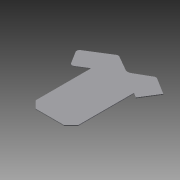
# Autodesk Inventor part: Boilermake_PCBMechanicalOverlay
Saved by Autodesk Inventor 2014 (Build 180170000, 170)
## iProperties
Created: 2014-09-13
Part Number: Boilermake_PCBMechanicalOverlay
Material: Generic
Document SubType Name: Modeling
Designer: Leeroy
Density: 1 g/cm^3
Appearance: Default
Author: Leeroy
Autodesk Inventor part; units mm, degrees
ref_plane "YZ Plane" through (0, 0, 0) normal (1, 0, 0) x (0, 1, 0)
ref_plane "XZ Plane" through (0, 0, 0) normal (0, 1, 0) x (-1, 0, 0)
ref_plane "XY Plane" through (0, 0, 0) normal (0, 0, 1) x (1, 0, 0)
sketch "Sketch1" plane through (0, 0, 0) normal (0, 0, 1) x (1, 0, 0)
  line L0 (19.7536, 18.501) -> (19.7536, -51.499)
  line L1 (-40.2464, -51.499) -> (-40.2464, 18.501)
  line L2 (-40.2464, -51.499) -> (-30.2464, -61.499)
  line L3 (-30.2464, -61.499) -> (9.7536, -61.499)
  line L4 (9.7536, -61.499) -> (19.7536, -51.499)
  line L5 (5.9033, -42.3953) -> (-35.9604, 24.6005)
  line L6 (-41.4722, 25.873) -> (-55.041, 17.3943)
  line L7 (-60.5529, 18.6668) -> (-71.151, 35.6275)
  line L8 (8.6592, -43.0315) -> (13.7475, -39.852)
  line L9 (14.3837, -37.0961) -> (-27.4799, 29.8997)
  line L10 (-26.2074, 35.4116) -> (-14.9119, 42.4698)
  line L11 (-15.0424, 49.3323) -> (-34.727, 60.6155)
  line L12 (-38.8359, 60.5374) -> (-69.8786, 41.1398)
  arc A0 (-34.727, 60.6155) -> (-38.8359, 60.5374) centre (-36.7162, 57.1452) ccw
  arc A1 (-14.9119, 42.4698) -> (-15.0424, 49.3323) centre (-17.0316, 45.8619) ccw
  arc A2 (-35.9604, 24.6005) -> (-41.4722, 25.873) centre (-39.3526, 22.4808) ccw
  arc A3 (-26.2074, 35.4116) -> (-27.4799, 29.8997) centre (-24.0877, 32.0194) ccw
  arc A4 (5.9033, -42.3953) -> (8.6592, -43.0315) centre (7.5994, -41.3354) ccw
  arc A5 (13.7475, -39.852) -> (14.3837, -37.0961) centre (12.6876, -38.1559) ccw
  line L13 (-26.3961, -42.3953) -> (15.4675, 24.6005)
  line L14 (20.9794, 25.873) -> (34.5482, 17.3943)
  line L15 (40.3411, 19.095) -> (50.6682, 35.6217)
  line L16 (-29.152, -43.0315) -> (-34.2403, -39.852)
  line L17 (-34.8766, -37.0961) -> (6.9871, 29.8997)
  line L18 (5.7136, 35.4098) -> (-5.5789, 42.4725)
  line L19 (-5.4504, 49.3323) -> (14.2435, 60.6103)
  line L20 (18.3431, 60.5374) -> (49.3859, 41.1397)
  arc A6 (18.3431, 60.5374) -> (14.2435, 60.6103) centre (16.2322, 57.1397) ccw
  arc A7 (-5.4504, 49.3323) -> (-5.5789, 42.4725) centre (-3.4579, 45.8638) ccw
  arc A8 (20.9794, 25.873) -> (15.4675, 24.6005) centre (18.8597, 22.4808) ccw
  arc A9 (6.9871, 29.8997) -> (5.7136, 35.4098) centre (3.5938, 32.0177) ccw
  arc A10 (-29.152, -43.0315) -> (-26.3961, -42.3953) centre (-28.0922, -41.3354) ccw
  arc A11 (-34.8766, -37.0961) -> (-34.2403, -39.852) centre (-33.1805, -38.1559) ccw
  arc A12 (-15.0424, 49.3323) -> (-5.4504, 49.3323) centre (-10.2464, 55.8144) ccw
  circle A13 centre (-10.2464, -7.115) radius 26
  circle A14 centre (-10.2464, -7.115) radius 20
  line L21 (-40.2464, 18.501) -> (-40.2464, 26.3797)
  line L22 (19.7536, 18.501) -> (19.7536, 26.3797)
  line L23 (-60.5529, 18.6668) -> (-60.5529, 18.6668)
  line L24 (-55.041, 17.3943) -> (-55.041, 17.3943)
  line L25 (-69.8786, 41.1398) -> (-69.8787, 41.1397)
  line L26 (-71.1513, 35.6278) -> (-71.151, 35.6275)
  arc A15 (-69.8787, 41.1397) -> (-71.1513, 35.6278) centre (-67.7591, 37.7475) ccw
  arc A16 (-60.5529, 18.6668) -> (-55.041, 17.3943) centre (-57.1607, 20.7865) ccw
  line L27 (49.3957, 41.1336) -> (49.3859, 41.1397)
  line L28 (50.6682, 35.6217) -> (50.6682, 35.6217)
  line L29 (34.5482, 17.3943) -> (34.5579, 17.3883)
  line L30 (40.3411, 19.095) -> (40.0698, 18.6608)
  arc A17 (34.5579, 17.3883) -> (40.0698, 18.6608) centre (36.6776, 20.7804) ccw
  arc A18 (50.6682, 35.6217) -> (49.3957, 41.1336) centre (47.276, 37.7414) ccw
  point P0 (0, 0)
  point P1 (-9.2464, 46.01)
  point P2 (-36.8049, 61.8065)
  point P3 (-20.4928, 0)
  point P4 (-11.243, 46.015)
  point P5 (16.3218, 61.8004)
  dimension "d0" = 70
  dimension "d1" = 135
  dimension "d2" = 135
  dimension "d3" = 10
  dimension "d4" = 10
  dimension "d5" = 40
  dimension "d6" = 10
  dimension "d7" = 85
  dimension "d8" = 24
  dimension "d9" = 24
  dimension "d10" = 28
  dimension "d11" = 43
  dimension "d13" = 2
  dimension "d14" = 31
  dimension "d15" = 32
  dimension "d19" = 70
  dimension "d21" = 52
  dimension "d22" = 40
  dimension "d43" = 8.0635
  dimension "d66" = 54.384
  dimension "d74" = 4
  dimension "d75" = 4
  dimension "d77" = 43
  dimension "d78" = 85
  dimension "d79" = 4
  constraints: 62 end point, 37 point on circle, 20 tangent, 19 centre point, 11 perpendicular, 9 point on line, 6 equal radius, 6 parallel, 3 collinear, 1 coincident, 1 vertical
  measures "d0" distance of L1.start L1.end
  measures "d1" angle of L1 L2
  measures "d2" angle of L4 L0
  measures "d3" horizontal distance of L1.start L2.end
  measures "d4" horizontal distance of L3.end L0.end
  measures "d5" distance of L2.end L3.end
  measures "d6" distance between parallel lines of L9 L5
  measures "d7" distance between parallel lines of L8 L6
  measures "d8" distance between parallel lines of L5 L7
  measures "d9" distance from line of point (-9.246, 46.01) L9
  measures "d10" distance between parallel lines of L12 L6
  measures "d11" distance from line of point (-36.805, 61.807) L7
  measures "d13" radius of A4
  measures "d14" distance from line of L1 point (-9.246, 46.01)
  measures "d15" angle of L1 L5
  measures "d19" distance of L0.start L0.end
  measures "d21" diameter of A13
  measures "d22" diameter of A14
  measures "d43" radius of A12
  measures "d66" distance from line of A13.centre L3
  measures "d74" radius of A3
  measures "d75" radius of A15
  measures "d77" distance from line of point (16.322, 61.8) L15
  measures "d78" distance between parallel lines of L16 L14
  measures "d79" radius of A17
extrude "Extrusion2" add sketch "Sketch1" along normal blind 1
sketch "Sketch11" plane through (0, 0, 1) normal (0, 0, 1) x (1, 0, 0)
  line L0 (40.0698, 18.6608) -> (50.6682, 35.6217) projected
  line L1 (-15.0424, 49.3323) -> (-34.727, 60.6155) projected
  arc A0 (-34.727, 60.6155) -> (-38.8359, 60.5374) centre (-36.7162, 57.1452) ccw projected
  line L2 (-38.8359, 60.5374) -> (-69.8787, 41.1397) projected
  arc A1 (-69.8787, 41.1397) -> (-71.1513, 35.6278) centre (-67.7591, 37.7475) ccw projected
  line L3 (-71.1513, 35.6278) -> (-60.5529, 18.6668) projected
  arc A2 (-60.5529, 18.6668) -> (-55.041, 17.3943) centre (-57.1607, 20.7865) ccw projected
  line L4 (-55.041, 17.3943) -> (-41.4722, 25.873) projected
  arc A3 (-40.2464, 26.3797) -> (-41.4722, 25.873) centre (-39.3526, 22.4808) ccw projected
  line L5 (-40.2464, 26.3797) -> (-40.2464, -51.499) projected
  line L6 (-40.2464, -51.499) -> (-30.2464, -61.499) projected
  line L7 (-30.2464, -61.499) -> (9.7536, -61.499) projected
  line L8 (9.7536, -61.499) -> (19.7536, -51.499) projected
  line L9 (19.7536, -51.499) -> (19.7536, 26.3797) projected
  arc A4 (20.9794, 25.873) -> (19.7536, 26.3797) centre (18.8597, 22.4808) ccw projected
  line L10 (20.9794, 25.873) -> (34.5579, 17.3883) projected
  arc A5 (34.5579, 17.3883) -> (40.0698, 18.6608) centre (36.6776, 20.7804) ccw projected
  line L11 (40.0698, 18.6608) -> (50.6682, 35.6217) projected
  arc A6 (50.6682, 35.6217) -> (49.3957, 41.1336) centre (47.276, 37.7414) ccw projected
  line L12 (49.3957, 41.1336) -> (18.3431, 60.5374) projected
  arc A7 (18.3431, 60.5374) -> (14.2435, 60.6103) centre (16.2322, 57.1397) ccw projected
  line L13 (14.2435, 60.6103) -> (-5.4504, 49.3323) projected
  arc A8 (-5.4504, 49.3323) -> (-5.9605, 48.9843) centre (-3.4579, 45.8638) ccw projected
  arc A9 (-14.528, 48.9816) -> (-5.9605, 48.9843) centre (-10.2464, 55.8144) ccw projected
  arc A10 (-14.528, 48.9816) -> (-15.0424, 49.3323) centre (-17.0316, 45.8619) ccw projected
  line L14 (41.5088, 46.0618) -> (26.6711, 22.3165)
  point P0 (0, 0)
  dimension "d80" = 13.3
  constraints: 2 end point, 2 point on line, 1 perpendicular
  measures "d80" distance between parallel lines of L0 L14
extrude "Extrusion9" cut sketch "Sketch11" against normal blind 10 contours A5 L10 L14 L12 A6 L0
body "Solid2"
